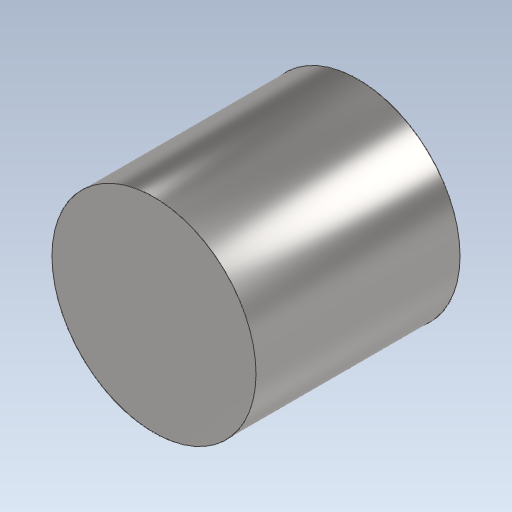
# Autodesk Inventor part: Neodymium_magnet_Phi3_T3
Saved by Autodesk Inventor 2020 (Build 240168000, 168)
## iProperties
Part Number: Neodymium_magnet_Phi3_T3
Material: 一般
Document SubType Name: Modeling
Designer: Masato Kubotera
Density: 1 g/cm^3
Appearance: 半つや出し
Description: ReadyMade
Catalog Web Link: https://www.amazon.co.jp/gp/product/B08Q3TWCHC/ref=ppx_yo_dt_b_asin_title_o08_s00?ie=UTF8&psc=1
Mass: 0.0212058 g
Surface Area: 0.424115 cm^2
Volume: 0.0212058 cm^3
Author: Masato Kubotera
Autodesk Inventor part; units mm, degrees
ref_plane "YZ Plane" through (0, 0, 0) normal (1, 0, 0) x (0, 1, 0)
ref_plane "XZ Plane" through (0, 0, 0) normal (0, 1, 0) x (-1, 0, 0)
ref_plane "XY Plane" through (0, 0, 0) normal (0, 0, 1) x (1, 0, 0)
sketch "スケッチ1" plane through (0, 0, 0) normal (0, 0, 1) x (1, 0, 0)
  circle A0 centre (0, 0) radius 1.5
  dimension "d0" = 3
  constraints: 1 centre point, 1 coincident
  measures "d0" diameter of A0
extrude "押し出し1" add sketch "スケッチ1" along normal blind 3
